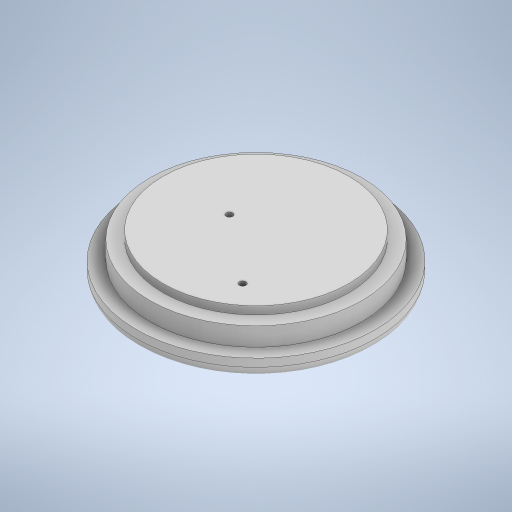
# Autodesk Inventor part: Cap
Saved by Autodesk Inventor 2024 (Build 280153000, 153)
## iProperties
Created: 2023-07-10
Part Number: Cap
Material: Generic
Document SubType Name: Modeling
Designer: westy
Density: 1 g/cm^3
Appearance: Default
Author: westy
Autodesk Inventor part; units mm, degrees
ref_plane "YZ Plane" through (0, 0, 0) normal (1, 0, 0) x (0, 1, 0)
ref_plane "XZ Plane" through (0, 0, 0) normal (0, 1, 0) x (-1, 0, 0)
ref_plane "XY Plane" through (0, 0, 0) normal (0, 0, 1) x (1, 0, 0)
sketch "Sketch1" plane through (0, 0, 0) normal (0, 1, 0) x (-1, 0, 0)
  circle A0 centre (0, 0) radius 40
  circle A1 centre (0, 0) radius 35
  dimension "d0" = 80
  dimension "d1" = 70
  constraints: 2 centre point, 2 coincident
  measures "d0" diameter of A0
  measures "d1" diameter of A1
extrude "Extrusion1" add sketch "Sketch1" along normal blind 10 contours A1
extrude "Extrusion2" add sketch "Sketch1" along normal blind 7
sketch "Sketch3" plane through (0, 0, 0) normal (0, -1, 0) x (1, 0, 0)
  circle A0 centre (0, 0) radius 45
  dimension "d14" = 90
  constraints: 1 centre point, 1 coincident
  measures "d14" diameter of A0
extrude "Extrusion4" add sketch "Sketch3" along normal blind 7
fillet "Fillet1" radius 4 1 edges at (-45, -7, 0)
sketch "Sketch4" plane through (0, 10, 0) normal (0, 1, 0) x (1, 0, 0)
  circle A0 centre (14.9762, -20.0178) radius 12
  circle A1 centre (-10, 0) radius 27
  circle A2 centre (14.9762, -20.0178) radius 1.25
  circle A3 centre (-10, 0) radius 1.25
  point P0 (0, 0)
  dimension "d24" = 24
  dimension "d25" = 54
  dimension "d26" = 10
  dimension "d27" = 2.5
  dimension "d28" = 2.5
  dimension "d31" = 25
  constraints: 4 centre point, 2 coincident
  measures "d24" diameter of A0
  measures "d25" diameter of A1
  measures "d26" distance of point (0, 0) A1.centre
  measures "d27" diameter of A2
  measures "d28" diameter of A3
  measures "d31" distance of point (0, 0) A0.centre
extrude "Extrusion5" cut sketch "Sketch4" against normal blind 5 contours A2 | A3
body "Solid1"
